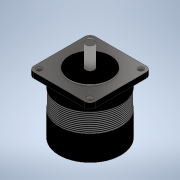
# Autodesk Inventor part: BLDC_motor
Saved by Autodesk Inventor 2020 (Build 240168000, 168)
## iProperties
Created: 2021-06-11
Part Number: BLDC_motor
Material: 一般
Document SubType Name: Modeling
Designer: user
Density: 1 g/cm^3
Appearance: 鋼 - 拋光
Author: user
Autodesk Inventor part; units mm, degrees
ref_plane "YZ Plane" through (0, 0, 0) normal (1, 0, 0) x (0, 1, 0)
ref_plane "XZ Plane" through (0, 0, 0) normal (0, 1, 0) x (-1, 0, 0)
ref_plane "XY Plane" through (0, 0, 0) normal (0, 0, 1) x (1, 0, 0)
sketch "草圖1" plane through (0, 0, 0) normal (0, 1, 0) x (-1, 0, 0)
  line L0 (23.5, 28.5) -> (-23.5, 28.5)
  line L1 (-28.5, 23.5) -> (-28.5, -23.5)
  line L2 (-23.5, -28.5) -> (23.5, -28.5)
  line L3 (28.5, -23.5) -> (28.5, 23.5)
  circle A0 centre (23.5, 23.5) radius 2.5
  circle A1 centre (23.5, -23.5) radius 2.5
  circle A2 centre (-23.5, -23.5) radius 2.5
  circle A3 centre (-23.5, 23.5) radius 2.5
  arc A4 (28.5, 23.5) -> (23.5, 28.5) centre (23.5, 23.5) ccw
  arc A5 (-23.5, 28.5) -> (-28.5, 23.5) centre (-23.5, 23.5) ccw
  arc A6 (-28.5, -23.5) -> (-23.5, -28.5) centre (-23.5, -23.5) ccw
  arc A7 (23.5, -28.5) -> (28.5, -23.5) centre (23.5, -23.5) ccw
  point P0 (0, 0)
  point P1 (28.5, 28.5)
  point P2 (-28.5, -28.5)
  point P3 (28.5, -28.5)
  dimension "d0" = 57
  dimension "d1" = 57
  dimension "d2" = 5
  dimension "d3" = 47
  dimension "d4" = 5
  dimension "d5" = 5
  dimension "d6" = 5
  dimension "d7" = 5
  dimension "d8" = 5
  dimension "d9" = 5
  dimension "d10" = 5
  dimension "d11" = 5
  dimension "d12" = 28.5
  dimension "d13" = 28.5
  constraints: 8 centre point, 8 end point, 8 point on circle, 8 tangent, 6 equal radius, 6 point on line, 2 parallel, 1 horizontal, 1 perpendicular
  measures "d0" distance of point (-28.5, -28.5) point (28.5, -28.5)
  measures "d1" distance of point (28.5, -28.5) point (28.5, 28.5)
  measures "d2" diameter of A0
  measures "d3" distance of A2.centre A1.centre
  measures "d4" distance from line of L1 A2.centre
  measures "d5" distance from line of L2 A1.centre
  measures "d6" distance from line of L2 A2.centre
  measures "d7" distance from line of L1 A3.centre
  measures "d8" distance from line of L0 A3.centre
  measures "d9" distance from line of L0 A0.centre
  measures "d10" distance from line of L3 A0.centre
  measures "d11" radius of A4
  measures "d12" distance from line of point (0, 0) L2
  measures "d13" distance from line of point (0, 0) L3
extrude "擠出1" add sketch "草圖1" along normal blind 5
sketch "草圖2" plane through (0, 5, 0) normal (0, 1, 0) x (1, 0, 0)
  circle A0 centre (0, 0) radius 19
  dimension "d16" = 38
  constraints: 1 centre point, 1 coincident
  measures "d16" diameter of A0
extrude "擠出2" add sketch "草圖2" along normal blind 1.2
sketch "草圖3" plane through (0, 6.2, 0) normal (0, 1, 0) x (1, 0, 0)
  circle A0 centre (0, 0) radius 4
  dimension "d19" = 8
  constraints: 1 centre point, 1 coincident
  measures "d19" diameter of A0
extrude "擠出3" add sketch "草圖3" along normal blind 20
sketch "草圖4" plane through (0, 26.2, 0) normal (0, 1, 0) x (1, 0, 0)
  line L0 (-1.8432, 3.55) -> (1.8432, 3.55)
  circle A0 centre (0, 0) radius 4 projected
  circle A1 centre (0, 0) radius 4 projected
  arc A2 (1.8432, 3.55) -> (-1.8432, 3.55) centre (0, 0) ccw
  line L1 (28.5, -23.5) -> (28.5, 23.5) projected
  point P0 (0, -4)
  dimension "d22" = 7.55
  dimension "d23" = 28.5
  constraints: 5 point on circle, 2 end point, 1 centre point, 1 coincident, 1 concentric, 1 horizontal
  measures "d22" distance from line of A1.start L0
  measures "d23" distance from line of L1 A1.start
extrude "擠出4" cut sketch "草圖4" against normal blind 15 contours A0 L0 picked at (-0.3162, 3.662)
sketch "草圖5" plane through (0, 0, 0) normal (0, -1, 0) x (1, 0, 0)
  circle A0 centre (0, 0) radius 28.5
  dimension "d26" = 57
  constraints: 1 centre point, 1 coincident
  measures "d26" diameter of A0
extrude "擠出5" add sketch "草圖5" along normal blind 9.25
sketch "草圖6" plane through (0, -9.25, 0) normal (0, -1, 0) x (1, 0, 0)
  circle A0 centre (0, 0) radius 28
  dimension "d29" = 56
  constraints: 1 centre point, 1 coincident
  measures "d29" diameter of A0
extrude "擠出6" add sketch "草圖6" along normal blind 17.5
sketch "草圖7" plane through (0, -26.75, 0) normal (0, -1, 0) x (1, 0, 0)
  circle A0 centre (0, 0) radius 4 projected
  circle A1 centre (0, 0) radius 28.5
  constraints: 1 centre point, 1 coincident
extrude "擠出7" add sketch "草圖7" along normal blind 23 contours A0 | A1
thread "螺紋1" size "M56x1.5" class "6g" standard "ANSI Metric M Profile" length 103
